Cam Halter 3 (Autodesk Fusion 360 design; units mm, degrees)
Autodesk Fusion 360 part; units mm, degrees
sketch "Sketch1" plane through (0, 0, 0) normal (0, 0, 1) x (1, 0, 0)
  circle A0 centre (0, 0) radius 3.7
  circle A1 centre (0, 0) radius 6
  line L0 (-25, -13.2) -> (25, -13.2)
  line L1 (25, -13.2) -> (25, -17.2)
  line L2 (25, -17.2) -> (-25, -17.2)
  line L3 (-25, -17.2) -> (-25, -13.2)
  line L4 (-6, 0) -> (6, 0)
  line L5 (6, 0) -> (6, -13.2)
  line L6 (6, -13.2) -> (-6, -13.2)
  line L7 (-6, -13.2) -> (-6, 0)
  point P0 (0, -13.2)
  dimension "d1" = 7.4
  dimension "d2" = 12
  dimension "d7" = 50
  dimension "d8" = 13.2
  dimension "d30" = 4
  constraint coincident A0.centre A1.centre
  constraint horizontal L0
  constraint vertical L1
  constraint horizontal L2
  constraint vertical L3
  constraint midpoint L0 P0
  constraint vertical A0.centre P0
  constraint horizontal L4
  constraint vertical L5
  constraint horizontal L6
  constraint vertical L7
  constraint collinear L0 L6
  constraint tangent A1 L7
  constraint tangent A1 L5
  constraint coincident A0.centre L4
  measures "d1" diameter of A0
  measures "d2" diameter of A1
  measures "d7" distance of L0.start L0.end
  measures "d8" distance of A0.centre L0
  measures "d30" distance of L0.start L2.end
extrude "Extrude1" add sketch "Sketch1" along normal blind 2 contours A0 L4 | A0 A1 L4 | A0 A1 L4 | A0 L4
extrude "Extrude2" add sketch "Sketch1" along normal blind 18 contours A0 A1 L4 | A0 A1 L4
extrude "Extrude3" add sketch "Sketch1" along normal blind 12 contours A1 L0 L5 L6 L7
extrude "Extrude4" add sketch "Sketch1" along normal blind 30 contours L0 L1 L2 L3 L6
sketch "Sketch4" plane through (0, -13.2, 0) normal (0, 1, 0) x (-1, 0, 0)
  line L0 (6, 12) -> (6, 0)
  line L1 (6, 0) -> (25, 0)
  line L2 (25, 0) -> (25, 30)
  line L3 (25, 30) -> (-25, 30)
  line L4 (-25, 30) -> (-25, 0)
  line L5 (-25, 0) -> (-6, 0)
  line L6 (-6, 0) -> (-6, 12)
  line L7 (-6, 12) -> (6, 12)
  circle A0 centre (-19, 15) radius 1.5
  circle A1 centre (19, 15) radius 1.5
  point P0 (-25, 15)
  point P1 (25, 15)
  dimension "d31" = 3
  dimension "d32" = 3
  dimension "d33" = 6
  dimension "d35" = 6
  constraint midpoint L4 P0
  constraint midpoint L2 P1
  constraint horizontal A0.centre P0
  constraint horizontal A1.centre P1
  measures "d31" diameter of A0
  measures "d32" diameter of A1
  measures "d33" distance of A0.centre P0
  measures "d35" distance of A1.centre P1
chamfer "Chamfer1" distance 2 distance2 30 1 edges at (0, -17.2, 0) measured on face at (-2, -4.4, 0)
extrude "Extrude8" cut sketch "Sketch4" against normal blind 16 contours A0 | A1
